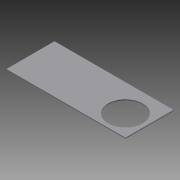
# Autodesk Inventor part: Bearing plate version 2.0
Saved by Autodesk Inventor 2015 (Build 190159000, 159)
## iProperties
Created: 2015-01-19
Part Number: Bearing plate version 2.0
Material: Generic
Document SubType Name: Modeling
Designer: chapale16
Density: 1 g/cm^3
Appearance: Default
Author: chapale16
Autodesk Inventor part; units mm, degrees
ref_plane "YZ Plane" through (0, 0, 0) normal (1, 0, 0) x (0, 1, 0)
ref_plane "XZ Plane" through (0, 0, 0) normal (0, 1, 0) x (-1, 0, 0)
ref_plane "XY Plane" through (0, 0, 0) normal (0, 0, 1) x (1, 0, 0)
sketch "Sketch1" plane through (0, 0, 0) normal (0, 1, 0) x (-1, 0, 0)
  line L0 (0, 0) -> (49.9643, 0)
  line L1 (0, -49.9643) -> (0, 0)
  line L2 (0, 0) -> (282.6258, 0)
  line L3 (282.6258, 0) -> (282.6258, -114.3)
  line L4 (282.6258, -114.3) -> (0, -114.3)
  line L5 (0, -114.3) -> (0, 0)
  circle A0 centre (49.9643, -49.9643) radius 40.9956
  dimension "d2" = 282.6258
  dimension "d3" = 114.3
  dimension "d4" = 81.9912
  constraints: 12 end point, 2 horizontal, 2 parallel, 1 centre point, 1 perpendicular
  measures "d2" distance of L3.end L4.end
  measures "d3" distance of L2.end L3.end
  measures "d4" diameter of A0
extrude "Extrusion1" add sketch "Sketch1" along normal blind 2.2098
body "Solid1"
